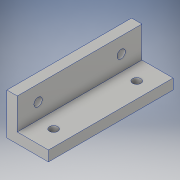
# Autodesk Inventor part: Beefy L
Saved by Autodesk Inventor 2018 (Build 220112000, 112)
## iProperties
Created: 2018-09-24
Part Number: Beefy L
Material: Aluminum 6061
Document SubType Name: Modeling
Designer: maste
Density: 2.7 g/cm^3
Appearance: Aluminum - Flat
Author: maste
Autodesk Inventor part; units mm, degrees
ref_plane "YZ Plane" through (0, 0, 0) normal (1, 0, 0) x (0, 1, 0)
ref_plane "XZ Plane" through (0, 0, 0) normal (0, 1, 0) x (-1, 0, 0)
ref_plane "XY Plane" through (0, 0, 0) normal (0, 0, 1) x (1, 0, 0)
sketch "Sketch1" plane through (0, 0, 0) normal (0, 0, 1) x (1, 0, 0)
  line L0 (0, 0) -> (25.4, 0)
  line L1 (25.4, 0) -> (25.4, 6.35)
  line L2 (25.4, 6.35) -> (0, 6.35)
  line L3 (0, 6.35) -> (0, 0)
  line L4 (0, 0) -> (6.35, 0)
  line L5 (6.35, 0) -> (6.35, 25.4)
  line L6 (6.35, 25.4) -> (0, 25.4)
  line L7 (0, 25.4) -> (0, 0)
  dimension "d0" = 25.4
  dimension "d1" = 6.35
  dimension "d2" = 6.35
  dimension "d3" = 25.4
  constraints: 16 end point, 4 parallel, 2 horizontal, 2 perpendicular
  measures "d0" distance of L2.end L1.end
  measures "d1" distance of L1.end L0.end
  measures "d2" distance of L6.end L5.end
  measures "d3" distance of L5.end L4.end
extrude "Extrusion1" add sketch "Sketch1" along normal blind 76.2
sketch "Sketch2" plane through (6.35, 6.35, 0) normal (0, 1, 0) x (1, 0, 0)
  line L0 (-6.35, 0) -> (19.05, 0) projected
  line L1 (19.05, 0) -> (0, 0)
  line L2 (9.525, 0) -> (9.525, -76.2)
  line L3 (-6.35, -76.2) -> (19.05, -76.2) projected
  line L4 (9.525, 0) -> (9.525, -12.7)
  line L5 (9.525, -76.2) -> (9.525, -63.5)
  circle A0 centre (9.525, -63.5) radius 2.54
  circle A1 centre (9.525, -12.7) radius 2.54
  dimension "d6" = 19.05
  dimension "d7" = 12.7
  dimension "d8" = 12.7
  dimension "d9" = 5.08
  dimension "d10" = 5.08
  constraints: 8 end point, 4 point on line, 2 centre point, 2 coincident, 1 midpoint, 1 vertical
  measures "d6" distance of L0.end L1.end
  measures "d7" distance of L2.start L4.end
  measures "d8" distance of L2.end L5.end
  measures "d9" diameter of A0
  measures "d10" diameter of A1
extrude "Extrusion2" cut sketch "Sketch2" against normal blind 25.4
sketch "Sketch3" plane through (6.35, 6.35, 0) normal (1, 0, 0) x (0, 0, -1)
  line L0 (0, 0) -> (0, 19.05) projected
  line L1 (0, 0) -> (0, 19.05)
  line L2 (0, 19.05) -> (0, 9.525)
  line L3 (0, 9.525) -> (-76.2, 9.525)
  line L4 (-76.2, 19.05) -> (-76.2, -6.35) projected
  line L5 (-76.2, 9.525) -> (-63.5, 9.525)
  line L6 (0, 9.525) -> (-12.7, 9.525)
  circle A0 centre (-63.5, 9.525) radius 2.54
  circle A1 centre (-12.7, 9.525) radius 2.54
  point P0 (0, -6.35)
  dimension "d13" = 12.7
  dimension "d14" = 12.7
  dimension "d15" = 5.08
  constraints: 10 end point, 3 point on line, 2 centre point, 2 coincident, 1 collinear, 1 midpoint, 1 perpendicular
  measures "d13" distance of L3.end L5.end
  measures "d14" distance of L2.end L6.end
  measures "d15" diameter of A0
extrude "Extrusion3" cut sketch "Sketch3" against normal blind 25.4
body "Solid1"
